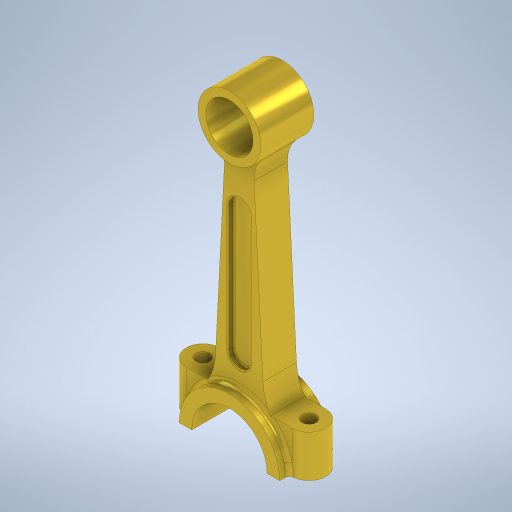
# Autodesk Inventor part: Part3 CONNECTING ROD
Saved by Autodesk Inventor 2023 (Build 270158000, 158)
## iProperties
Created: 2025-10-01
Part Number: Part3 CONNECTING ROD
Material: Stainless Steel
Document SubType Name: Sheet Metal
Designer: ayush
Density: 8 g/cm^3
Sheet Metal Rule: Default_mm
Appearance: Metal 2400F Hot
Author: ayush
Autodesk Inventor part; units mm, degrees
ref_plane "YZ Plane" through (0, 0, 0) normal (1, 0, 0) x (0, 1, 0)
ref_plane "XZ Plane" through (0, 0, 0) normal (0, 1, 0) x (-1, 0, 0)
sketch "Sketch1" plane through (0, 0, 0) normal (0, 0, 1) x (1, 0, 0)
  circle A0 centre (0, 75.2152) radius 22.5
  circle A1 centre (0, 75.2152) radius 16.9
  arc A2 (36, -125.9848) -> (-36, -125.9848) centre (0, -125.9848) ccw
  arc A3 (27, -125.9848) -> (-27, -125.9848) centre (0, -125.9848) ccw
  line L0 (-10, 55.0596) -> (-17.8497, -94.7216)
  line L1 (0, 75.2152) -> (0, -125.9848) construction
  line L2 (10, 55.0596) -> (17.8497, -94.7216)
  line L3 (-36, -125.9848) -> (-27, -125.9848)
  line L4 (27, -125.9848) -> (36, -125.9848)
  point P0 (0, 0)
  dimension "d1" = 45
  dimension "d0" = 33.8
  dimension "d2" = 72
  dimension "d3" = 54
  dimension "d4" = 201.2
  dimension "d5" = 10
  dimension "d6" = 3
  constraints: 10 end point, 5 point on circle, 3 centre point, 2 coincident, 2 horizontal, 2 symmetric about line, 1 vertical, 3 other
  measures "d0" diameter of A1
  measures "d2" diameter of A2
  measures "d3" diameter of A3
  measures "d4" distance of point (0, 75.215) A2.centre
  measures "d5" distance from line of L1 L0.start
  measures "d6" angle of L1 L0
extrude "Extrusion1" add sketch "Sketch1" along normal mid plane 38 contours A0 | A2 L4 A3 L3
extrude "Extrusion2" add sketch "Sketch1" along normal mid plane 24 contours A0 L2 A2 L0
fillet "Fillet1" radius 40 2 edges at (17.8497, -94.7216, 0) (-17.8497, -94.7216, 0)
fillet "Fillet2" radius 22 2 edges at (-10, 55.0596, 0) (10, 55.0596, 0)
sketch "Sketch2" plane through (0, 0, 12) normal (0, 0, 1) x (1, 0, 0)
  line L0 (0, 19.6152) -> (0, -70.3848) construction
  line L1 (-8, 19.6152) -> (-8, -70.3848)
  line L2 (8, -70.3848) -> (8, 19.6152)
  arc A0 (8, 19.6152) -> (-8, 19.6152) centre (0, 19.6152) ccw
  arc A1 (-8, -70.3848) -> (8, -70.3848) centre (0, -70.3848) ccw
  circle A2 centre (0, 75.2152) radius 16.9 construction
  point P0 (0, 0)
  point P1 (0, -25.3848)
  dimension "d13" = 8
  dimension "d15" = 90
  dimension "d16" = 55.6
  constraints: 8 end point, 4 point on circle, 4 tangent, 2 centre point, 1 midpoint, 1 parallel, 1 vertical, 1 vertical alignment
  measures "d13" radius of A0
  measures "d15" distance of L0.end L0.start
  measures "d16" distance of L0.start A2.centre
extrude "Extrusion3" cut sketch "Sketch2" against normal blind 4
mirror "Mirror1" about plane through (0, 0, 0) normal (0, 0, 1) of "Extrusion3"
fillet "Fillet3" radius 1 16 edges at (0, 27.6152, 12) (8, -25.3848, 12) (0, -78.3848, 12) (-8, -25.3848, 12) (0, 27.6152, 8) (8, -25.3848, 8) (0, -78.3848, 8) (-8, -25.3848, 8) (0, 27.6152, -12) (-8, -25.3848, -12) (0, -78.3848, -12) (8, -25.3848, -12) (0, -78.3848, -8) (-8, -25.3848, -8) (0, 27.6152, -8) (8, -25.3848, -8)
ref_plane "Work Plane1" through (27, -95.9848, 19) normal (0, -1, 0) x (1, 0, 0)
sketch "Sketch3" plane through (27, -95.9848, 19) normal (0, -1, 0) x (1, 0, 0)
  line L0 (-54, 0) -> (0, 0) construction
  line L1 (9, 0) -> (9, -38) construction
  line L2 (11, -19) -> (-65, -19) construction
  line L3 (-4.5, -38) -> (-4.5, 0) construction
  line L4 (11, -31) -> (-65, -31)
  line L5 (-65, -7) -> (11, -7)
  arc A0 (11, -31) -> (11, -7) centre (11, -19) ccw
  arc A1 (-65, -7) -> (-65, -31) centre (-65, -19) ccw
  line L6 (-27, -19) -> (-27, 37.5868) construction
  dimension "d21" = 12
  dimension "d22" = 76
  constraints: 10 end point, 4 point on circle, 4 tangent, 2 centre point, 1 coincident, 1 midpoint, 1 parallel, 1 perpendicular, 1 vertical
  measures "d21" radius of A0
  measures "d22" distance of L2.start L2.end
extrude "Extrusion4" add sketch "Sketch3" along normal up to surface (30 mm away)
sketch "Sketch4" plane through (0, 0, 0) normal (0, 0, 1) x (1, 0, 0)
  arc A0 (27, -125.9848) -> (-27, -125.9848) centre (0, -125.9848) ccw projected
  line L0 (-27, -125.9848) -> (27, -125.9848) projected
  point P0 (0, 0)
extrude "Extrusion5" cut sketch "Sketch4" along normal through all both and the other way through all
sketch "Sketch5" plane through (27, -125.9848, -19) normal (0, -1, 0) x (1, 0, 0)
  arc A0 (-65, 31) -> (-65, 7) centre (-65, 19) ccw projected
  point P0 (-27, 19)
  constraints: 1 coincident
hole "Hole1" at (-38, -125.9848, 0) direction (0, 1, 0) diameter 10 end through all
sketch "Sketch6" plane through (27, -125.9848, -19) normal (0, -1, 0) x (1, 0, 0)
  arc A0 (11, 7) -> (11, 31) centre (11, 19) ccw projected
  point P0 (-27, 19)
  constraints: 1 coincident
hole "Hole2" at (38, -125.9848, 0) direction (0, 1, 0) diameter 10 end through all
fillet "Fillet4" radius 3 2 edges at (0, -89.9848, 12) (0, -89.9848, -12)
equation "\"d32\" = Thickness"
equation "\"BendRadius\" = Thickness"
equation "\"BendReliefWidth\" = Thickness"
equation "\"BendReliefDepth\" = 0.5 * Thickness"
equation "\"CornerReliefSize\" = 4 * Thickness"
equation "\"MinimumRemnant\" = 2 * Thickness"
equation "\"TransitionRadius\" = BendRadius"
equation "\"JacobiRadiusSize\" = BendRadius"
equation "\"GapSize\" = Thickness"
equation "\"Thickness\" = 0.5"
body "Solid1"
